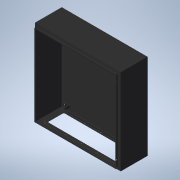
# Autodesk Inventor part: 1060.000(2)_P1
Saved by Autodesk Inventor 2021 (Build 250183000, 183)
## iProperties
Created: 2025-09-22
Part Number: 1060.000(2)_P1
Material: Generic
Catalog Web Link: www.cadenas.de
Description: AE 2.0 Gehaeuse-AE 2.0 Gehaeuse
Vendor: RITTAL
Document SubType Name: Modeling
Designer: psAdmin
Manufacturer: RITTAL
Mass: 1295.88 g
Surface Area: 17146.7 cm^2
Volume: 1295.88 cm^3
Density: 1 g/cm^3
Appearance: PSOLRGB-176-176-176
Category: PARTsolutions
Company: RITTAL
Title: 1060.000(2)_P1
Author: Cadenas PARTsolutions
Comments: AE 2.0 Gehaeuse
PSOL_IDENT_0: {$CADENAS_DATA/23d-libs/rittal/schaltschranksys/kompakt_schaltschr/parts_ae_2_0/gehaeuse_ae_2_0.prj}
PSOL_IDENT_1: ,190 {VTYP=3D},{NB=1060.000(2)_P1},{LINA=1060.000(2)_P1},{NN=AE 2.0 Gehaeuse},{DATE=25.07.2025 12:41
PSOL_IDENT_2: :23},{GEOMDATE=24.07.2025 05:50:00},{VERSION=},{LINEID=350},{WBVAR=DETAIL},{WBNUMERIC=DETAIL}  {NB=1
PSOL_IDENT_3: 060.000(2)_P1},{LINA=1060.000(2)_P1},{KT=DUMMY},{DETAIL=2},{BEZ1=Neues Kompaktgehäuse},{BEZ2=Stahlbl
PSOL_IDENT_4: ech},{BEZ3=eintürig},{TUER=1},{B=600},{H=600},{T=210},{F=550},{G=575},{B1=600},{BEST=1060.000},{B3=5
PSOL_IDENT_5: 60.000},{B4=470.000},{B5=498.000},{BB5=0.000},{H1=600},{H3=560.000},{H4=85.000},{H5=113.000},{HH5=4.
PSOL_IDENT_6: 000},{T5=93.500},{R1=31.000},{R2=8.000},{T1=210},{F1=550},{G1=575},{VERS3=0},{VERS=7},{CNSECLASS51=2
PSOL_IDENT_7: 7-18-01-02},{CNSECLASS70=27-18-01-01},{CNSECLASS80=27-18-01-01},{CNSETIM40=EC000261},{S=1.50},{W=600
PSOL_IDENT_8: .000},{W1=556.000},{W2=500.000},{HH=600.000},{HH1=556.000},{HH2=550.000},{HH3=475.000},{D=187.500},{
PSOL_IDENT_9: D1=205.100},{VERS1=1},{GEW=22,3},{CNSETIM80=EC000261},{CNSETIM90=EC000261},{CNSECLASS60=27-18-01-01}
PSOL_IDENT_10: ,{UNSPSC=31-26-15-02}
NB: 1060.000(2)_P1
NN: AE 2.0 Gehaeuse
NT: AE 2.0 Gehaeuse
NBSYN: $BEST.($DETAIL.)_P1
LINA: 1060.000(2)_P1
CATALOG: Rittal
DETAIL: niedrig
BEZ1: Neues Kompaktgehäuse
BEZ2: Stahlblech
BEZ3: eintürig
TUER: 1
B: 600
H: 600
T: 210
F: 550
G: 575
B1: 600
BEST: 1060.000
B3: 560
B4: 470
B5: 498
BB5: 0
H1: 600
H3: 560
H4: 85
H5: 113
HH5: 4
T5: 93.5
R1: 31
R2: 8
T1: 210
F1: 550
G1: 575
VERS3: 0
VERS: 7
CNSECLASS70: 27-18-01-01
CNSECLASS80: 27-18-01-01
S: 1.5
W: 600
W1: 556
W2: 500
HH: 600
HH1: 556
HH2: 550
HH3: 475
D: 187.5
D1: 205.1
VERS1: 1
GEW: 22,3
CNSETIM80: EC000261
CNSETIM90: EC000261
CNSECLASS60: 27-18-01-01
UNSPSC: 31-26-15-02
SUPPLIER: RITTAL
ARTICLENO: 1060.000(2)_P1
BOMINFO: 1060.000(2)_P1
CREATOR: CADENAS GmbH
Autodesk Inventor part; units mm, degrees
(part 1 of 2)
sketch "Sketch_1" plane through (0, 0, 0) normal (0, 1, 0) x (1, 0, 0)
  line L0 (-300, -82.5) -> (300, -82.5)
  line L1 (300, -82.5) -> (300, 105)
  line L2 (300, 105) -> (-300, 105)
  line L3 (-300, 105) -> (-300, -82.5)
  line L4 (-298.5, -81) -> (298.5, -81)
  line L5 (298.5, -81) -> (298.5, 103.5)
  line L6 (298.5, 103.5) -> (-298.5, 103.5)
  line L7 (-298.5, 103.5) -> (-298.5, -81)
  constraints: 16 end point
extrude "Extrusion1" add sketch "Sketch_1" along normal blind 600
sketch "Sketch_2" plane through (0, 0, 82.5) normal (0, 0, 1) x (1, 0, 0)
  line L0 (-281, 19) -> (281, 19)
  line L1 (281, 19) -> (281, 581)
  line L2 (281, 581) -> (-281, 581)
  line L3 (-281, 581) -> (-281, 19)
  constraints: 8 end point
extrude "Extrusion2" cut sketch "Sketch_2" against normal blind 1.5
sketch "Sketch_3" plane through (0, 0, 0) normal (1, 0, 0) x (0, 0, -1)
  line L0 (-82.5, 590) -> (-81, 590)
  line L1 (-81, 590) -> (-81, 598.5)
  line L2 (-81, 598.5) -> (103.5, 598.5)
  line L3 (103.5, 598.5) -> (103.5, 1.5)
  line L4 (103.5, 1.5) -> (-81, 1.5)
  line L5 (-81, 1.5) -> (-81, 10)
  line L6 (-81, 10) -> (-82.5, 10)
  line L7 (-82.5, 10) -> (-82.5, 0)
  line L8 (-82.5, 0) -> (105, 0)
  line L9 (105, 0) -> (105, 600)
  line L10 (105, 600) -> (-82.5, 600)
  line L11 (-82.5, 600) -> (-82.5, 590)
  constraints: 24 end point
extrude "Extrusion3" add sketch "Sketch_3" along normal mid plane 600
sketch "Sketch_48" plane through (0, 0, -105) normal (0, 0, 1) x (1, 0, 0)
  line L0 (-295.5, 595.5) -> (-295.5, 4.5)
  line L1 (-295.5, 4.5) -> (295.5, 4.5)
  line L2 (295.5, 4.5) -> (295.5, 595.5)
  line L3 (295.5, 595.5) -> (-295.5, 595.5)
  constraints: 8 end point
extrude "Extrusion4" cut sketch "Sketch_48" along normal blind 1.5
sketch "Sketch_49" plane through (0, 0, -105) normal (0, 0, 1) x (1, 0, 0)
  line L0 (-295.5, 595.5) -> (-295.5, 4.5)
  line L1 (-295.5, 4.5) -> (295.5, 4.5)
  line L2 (295.5, 4.5) -> (295.5, 595.5)
  line L3 (295.5, 595.5) -> (-295.5, 595.5)
  line L4 (268.5, 8.5) -> (291.5, 8.5)
  line L5 (291.5, 8.5) -> (291.5, 31.5)
  line L6 (291.5, 31.5) -> (268.5, 31.5)
  line L7 (268.5, 31.5) -> (268.5, 8.5)
  line L8 (268.5, 568.5) -> (291.5, 568.5)
  line L9 (291.5, 568.5) -> (291.5, 591.5)
  line L10 (291.5, 591.5) -> (268.5, 591.5)
  line L11 (268.5, 591.5) -> (268.5, 568.5)
  line L12 (-291.5, 8.5) -> (-268.5, 8.5)
  line L13 (-268.5, 8.5) -> (-268.5, 31.5)
  line L14 (-268.5, 31.5) -> (-291.5, 31.5)
  line L15 (-291.5, 31.5) -> (-291.5, 8.5)
  line L16 (-291.5, 568.5) -> (-268.5, 568.5)
  line L17 (-268.5, 568.5) -> (-268.5, 591.5)
  line L18 (-268.5, 591.5) -> (-291.5, 591.5)
  line L19 (-291.5, 591.5) -> (-291.5, 568.5)
  constraints: 40 end point
extrude "Extrusion5" add sketch "Sketch_49" along normal blind 1.5
sketch "Sketch_50" plane through (0, 20, 0) normal (0, 1, 0) x (1, 0, 0)
  line L0 (-291.5, 103.5) -> (-290.1732, 103.5)
  line L1 (-290.1732, 103.5) -> (-289.0185, 101.5)
  line L2 (-289.0185, 101.5) -> (-270.9815, 101.5)
  line L3 (-270.9815, 101.5) -> (-269.8268, 103.5)
  line L4 (-269.8268, 103.5) -> (-268.5, 103.5)
  line L5 (-268.5, 103.5) -> (-268.5, 105)
  line L6 (-268.5, 105) -> (-270, 105)
  line L7 (-270, 105) -> (-271.1547, 103)
  line L8 (-271.1547, 103) -> (-288.8453, 103)
  line L9 (-288.8453, 103) -> (-290, 105)
  line L10 (-290, 105) -> (-291.5, 105)
  line L11 (-291.5, 105) -> (-291.5, 103.5)
  constraints: 24 end point
extrude "Extrusion6" add sketch "Sketch_50" along normal mid plane 15.35
sketch "Sketch_51" plane through (0, 20, 0) normal (0, 1, 0) x (1, 0, 0)
  line L0 (268.5, 103.5) -> (269.8268, 103.5)
  line L1 (269.8268, 103.5) -> (270.9815, 101.5)
  line L2 (270.9815, 101.5) -> (289.0185, 101.5)
  line L3 (289.0185, 101.5) -> (290.1732, 103.5)
  line L4 (290.1732, 103.5) -> (291.5, 103.5)
  line L5 (291.5, 103.5) -> (291.5, 105)
  line L6 (291.5, 105) -> (290, 105)
  line L7 (290, 105) -> (288.8453, 103)
  line L8 (288.8453, 103) -> (271.1547, 103)
  line L9 (271.1547, 103) -> (270, 105)
  line L10 (270, 105) -> (268.5, 105)
  line L11 (268.5, 105) -> (268.5, 103.5)
  constraints: 24 end point
extrude "Extrusion7" add sketch "Sketch_51" along normal mid plane 15.35
sketch "Sketch_52" plane through (0, 27.675, 0) normal (0, 1, 0) x (1, 0, 0)
  line L0 (-272.325, 101.5) -> (-272.325, 103)
  line L1 (-272.325, 103) -> (-271.1547, 103)
  line L2 (-271.1547, 103) -> (-270, 105)
  line L3 (-270, 105) -> (-265.5, 105)
  line L4 (-265.5, 105) -> (-265.5, 103.5)
  line L5 (-265.5, 103.5) -> (-269.8268, 103.5)
  line L6 (-269.8268, 103.5) -> (-270.9815, 101.5)
  line L7 (-270.9815, 101.5) -> (-272.325, 101.5)
  line L8 (-272.325, 101.5) -> (-272.325, 103)
  constraints: 18 end point
revolve "Revolution1" add sketch "Sketch_52" angle 90 about axis through (-272.325, 27.675, -101.5) along (0, 0, 1)
sketch "Sketch_53" plane through (0, 27.675, 0) normal (0, 1, 0) x (1, 0, 0)
  line L0 (-287.675, 103) -> (-287.675, 101.5)
  line L1 (-287.675, 101.5) -> (-289.0185, 101.5)
  line L2 (-289.0185, 101.5) -> (-290.1732, 103.5)
  line L3 (-290.1732, 103.5) -> (-294.5, 103.5)
  line L4 (-294.5, 103.5) -> (-294.5, 105)
  line L5 (-294.5, 105) -> (-290, 105)
  line L6 (-290, 105) -> (-288.8453, 103)
  line L7 (-288.8453, 103) -> (-287.675, 103)
  line L8 (-287.675, 103) -> (-287.675, 101.5)
  constraints: 18 end point
revolve "Revolution2" add sketch "Sketch_53" angle 90 about axis through (-287.675, 27.675, -103) along (0, 0, -1)
sketch "Sketch_54" plane through (0, 27.675, 0) normal (0, 1, 0) x (1, 0, 0)
  line L0 (287.675, 101.5) -> (287.675, 103)
  line L1 (287.675, 103) -> (288.8453, 103)
  line L2 (288.8453, 103) -> (290, 105)
  line L3 (290, 105) -> (294.5, 105)
  line L4 (294.5, 105) -> (294.5, 103.5)
  line L5 (294.5, 103.5) -> (290.1732, 103.5)
  line L6 (290.1732, 103.5) -> (289.0185, 101.5)
  line L7 (289.0185, 101.5) -> (287.675, 101.5)
  line L8 (287.675, 101.5) -> (287.675, 103)
  constraints: 18 end point
revolve "Revolution3" add sketch "Sketch_54" angle 90 about axis through (287.675, 27.675, -101.5) along (0, 0, 1)
sketch "Sketch_55" plane through (0, 27.675, 0) normal (0, 1, 0) x (1, 0, 0)
  line L0 (272.325, 103) -> (272.325, 101.5)
  line L1 (272.325, 101.5) -> (270.9815, 101.5)
  line L2 (270.9815, 101.5) -> (269.8268, 103.5)
  line L3 (269.8268, 103.5) -> (265.5, 103.5)
  line L4 (265.5, 103.5) -> (265.5, 105)
  line L5 (265.5, 105) -> (270, 105)
  line L6 (270, 105) -> (271.1547, 103)
  line L7 (271.1547, 103) -> (272.325, 103)
  line L8 (272.325, 103) -> (272.325, 101.5)
  constraints: 18 end point
revolve "Revolution4" add sketch "Sketch_55" angle 90 about axis through (272.325, 27.675, -103) along (0, 0, -1)
sketch "Sketch_56" plane through (0, 12.325, 0) normal (0, 1, 0) x (1, 0, 0)
  line L0 (-272.325, 101.5) -> (-272.325, 103)
  line L1 (-272.325, 103) -> (-271.1547, 103)
  line L2 (-271.1547, 103) -> (-270, 105)
  line L3 (-270, 105) -> (-265.5, 105)
  line L4 (-265.5, 105) -> (-265.5, 103.5)
  line L5 (-265.5, 103.5) -> (-269.8268, 103.5)
  line L6 (-269.8268, 103.5) -> (-270.9815, 101.5)
  line L7 (-270.9815, 101.5) -> (-272.325, 101.5)
  line L8 (-272.325, 101.5) -> (-272.325, 103)
  constraints: 18 end point
revolve "Revolution5" add sketch "Sketch_56" angle 90 about axis through (-272.325, 12.325, -101.5) along (0, 0, -1)
sketch "Sketch_57" plane through (0, 12.325, 0) normal (0, 1, 0) x (1, 0, 0)
  line L0 (-287.675, 103) -> (-287.675, 101.5)
  line L1 (-287.675, 101.5) -> (-289.0185, 101.5)
  line L2 (-289.0185, 101.5) -> (-290.1732, 103.5)
  line L3 (-290.1732, 103.5) -> (-294.5, 103.5)
  line L4 (-294.5, 103.5) -> (-294.5, 105)
  line L5 (-294.5, 105) -> (-290, 105)
  line L6 (-290, 105) -> (-288.8453, 103)
  line L7 (-288.8453, 103) -> (-287.675, 103)
  line L8 (-287.675, 103) -> (-287.675, 101.5)
  constraints: 18 end point
revolve "Revolution6" add sketch "Sketch_57" angle 90 about axis through (-287.675, 12.325, -103) along (0, 0, 1)
sketch "Sketch_58" plane through (0, 12.325, 0) normal (0, 1, 0) x (1, 0, 0)
  line L0 (287.675, 101.5) -> (287.675, 103)
  line L1 (287.675, 103) -> (288.8453, 103)
  line L2 (288.8453, 103) -> (290, 105)
  line L3 (290, 105) -> (294.5, 105)
  line L4 (294.5, 105) -> (294.5, 103.5)
  line L5 (294.5, 103.5) -> (290.1732, 103.5)
  line L6 (290.1732, 103.5) -> (289.0185, 101.5)
  line L7 (289.0185, 101.5) -> (287.675, 101.5)
  line L8 (287.675, 101.5) -> (287.675, 103)
  constraints: 18 end point
revolve "Revolution7" add sketch "Sketch_58" angle 90 about axis through (287.675, 12.325, -101.5) along (0, 0, -1)
sketch "Sketch_59" plane through (0, 12.325, 0) normal (0, 1, 0) x (1, 0, 0)
  line L0 (272.325, 103) -> (272.325, 101.5)
  line L1 (272.325, 101.5) -> (270.9815, 101.5)
  line L2 (270.9815, 101.5) -> (269.8268, 103.5)
  line L3 (269.8268, 103.5) -> (265.5, 103.5)
  line L4 (265.5, 103.5) -> (265.5, 105)
  line L5 (265.5, 105) -> (270, 105)
  line L6 (270, 105) -> (271.1547, 103)
  line L7 (271.1547, 103) -> (272.325, 103)
  line L8 (272.325, 103) -> (272.325, 101.5)
  constraints: 18 end point
revolve "Revolution8" add sketch "Sketch_59" angle 90 about axis through (272.325, 12.325, -103) along (0, 0, 1)
sketch "Sketch_60" plane through (0, 580, 0) normal (0, 1, 0) x (1, 0, 0)
  line L0 (-291.5, 103.5) -> (-290.1732, 103.5)
  line L1 (-290.1732, 103.5) -> (-289.0185, 101.5)
  line L2 (-289.0185, 101.5) -> (-270.9815, 101.5)
  line L3 (-270.9815, 101.5) -> (-269.8268, 103.5)
  line L4 (-269.8268, 103.5) -> (-268.5, 103.5)
  line L5 (-268.5, 103.5) -> (-268.5, 105)
  line L6 (-268.5, 105) -> (-270, 105)
  line L7 (-270, 105) -> (-271.1547, 103)
  line L8 (-271.1547, 103) -> (-288.8453, 103)
  line L9 (-288.8453, 103) -> (-290, 105)
  line L10 (-290, 105) -> (-291.5, 105)
  line L11 (-291.5, 105) -> (-291.5, 103.5)
  constraints: 24 end point
extrude "Extrusion8" add sketch "Sketch_60" along normal mid plane 15.35
sketch "Sketch_61" plane through (0, 580, 0) normal (0, 1, 0) x (1, 0, 0)
  line L0 (268.5, 103.5) -> (269.8268, 103.5)
  line L1 (269.8268, 103.5) -> (270.9815, 101.5)
  line L2 (270.9815, 101.5) -> (289.0185, 101.5)
  line L3 (289.0185, 101.5) -> (290.1732, 103.5)
  line L4 (290.1732, 103.5) -> (291.5, 103.5)
  line L5 (291.5, 103.5) -> (291.5, 105)
  line L6 (291.5, 105) -> (290, 105)
  line L7 (290, 105) -> (288.8453, 103)
  line L8 (288.8453, 103) -> (271.1547, 103)
  line L9 (271.1547, 103) -> (270, 105)
  line L10 (270, 105) -> (268.5, 105)
  line L11 (268.5, 105) -> (268.5, 103.5)
  constraints: 24 end point
extrude "Extrusion9" add sketch "Sketch_61" along normal mid plane 15.35
sketch "Sketch_62" plane through (0, 587.675, 0) normal (0, 1, 0) x (1, 0, 0)
  line L0 (-272.325, 101.5) -> (-272.325, 103)
  line L1 (-272.325, 103) -> (-271.1547, 103)
  line L2 (-271.1547, 103) -> (-270, 105)
  line L3 (-270, 105) -> (-265.5, 105)
  line L4 (-265.5, 105) -> (-265.5, 103.5)
  line L5 (-265.5, 103.5) -> (-269.8268, 103.5)
  line L6 (-269.8268, 103.5) -> (-270.9815, 101.5)
  line L7 (-270.9815, 101.5) -> (-272.325, 101.5)
  line L8 (-272.325, 101.5) -> (-272.325, 103)
  constraints: 18 end point
revolve "Revolution9" add sketch "Sketch_62" angle 90 about axis through (-272.325, 587.675, -101.5) along (0, 0, 1)
sketch "Sketch_63" plane through (0, 587.675, 0) normal (0, 1, 0) x (1, 0, 0)
  line L0 (-287.675, 103) -> (-287.675, 101.5)
  line L1 (-287.675, 101.5) -> (-289.0185, 101.5)
  line L2 (-289.0185, 101.5) -> (-290.1732, 103.5)
  line L3 (-290.1732, 103.5) -> (-294.5, 103.5)
  line L4 (-294.5, 103.5) -> (-294.5, 105)
  line L5 (-294.5, 105) -> (-290, 105)
  line L6 (-290, 105) -> (-288.8453, 103)
  line L7 (-288.8453, 103) -> (-287.675, 103)
  line L8 (-287.675, 103) -> (-287.675, 101.5)
  constraints: 18 end point
revolve "Revolution10" add sketch "Sketch_63" angle 90 about axis through (-287.675, 587.675, -103) along (0, 0, -1)
sketch "Sketch_64" plane through (0, 587.675, 0) normal (0, 1, 0) x (1, 0, 0)
  line L0 (287.675, 101.5) -> (287.675, 103)
  line L1 (287.675, 103) -> (288.8453, 103)
  line L2 (288.8453, 103) -> (290, 105)
  line L3 (290, 105) -> (294.5, 105)
  line L4 (294.5, 105) -> (294.5, 103.5)
  line L5 (294.5, 103.5) -> (290.1732, 103.5)
  line L6 (290.1732, 103.5) -> (289.0185, 101.5)
  line L7 (289.0185, 101.5) -> (287.675, 101.5)
  line L8 (287.675, 101.5) -> (287.675, 103)
  constraints: 18 end point
revolve "Revolution11" add sketch "Sketch_64" angle 90 about axis through (287.675, 587.675, -101.5) along (0, 0, 1)
sketch "Sketch_65" plane through (0, 587.675, 0) normal (0, 1, 0) x (1, 0, 0)
  line L0 (272.325, 103) -> (272.325, 101.5)
  line L1 (272.325, 101.5) -> (270.9815, 101.5)
  line L2 (270.9815, 101.5) -> (269.8268, 103.5)
  line L3 (269.8268, 103.5) -> (265.5, 103.5)
  line L4 (265.5, 103.5) -> (265.5, 105)
  line L5 (265.5, 105) -> (270, 105)
  line L6 (270, 105) -> (271.1547, 103)
  line L7 (271.1547, 103) -> (272.325, 103)
  line L8 (272.325, 103) -> (272.325, 101.5)
  constraints: 18 end point
revolve "Revolution12" add sketch "Sketch_65" angle 90 about axis through (272.325, 587.675, -103) along (0, 0, -1)
sketch "Sketch_66" plane through (0, 572.325, 0) normal (0, 1, 0) x (1, 0, 0)
  line L0 (-272.325, 101.5) -> (-272.325, 103)
  line L1 (-272.325, 103) -> (-271.1547, 103)
  line L2 (-271.1547, 103) -> (-270, 105)
  line L3 (-270, 105) -> (-265.5, 105)
  line L4 (-265.5, 105) -> (-265.5, 103.5)
  line L5 (-265.5, 103.5) -> (-269.8268, 103.5)
  line L6 (-269.8268, 103.5) -> (-270.9815, 101.5)
  line L7 (-270.9815, 101.5) -> (-272.325, 101.5)
  line L8 (-272.325, 101.5) -> (-272.325, 103)
  constraints: 18 end point
revolve "Revolution13" add sketch "Sketch_66" angle 90 about axis through (-272.325, 572.325, -101.5) along (0, 0, -1)
sketch "Sketch_67" plane through (0, 572.325, 0) normal (0, 1, 0) x (1, 0, 0)
  line L0 (-287.675, 103) -> (-287.675, 101.5)
  line L1 (-287.675, 101.5) -> (-289.0185, 101.5)
  line L2 (-289.0185, 101.5) -> (-290.1732, 103.5)
  line L3 (-290.1732, 103.5) -> (-294.5, 103.5)
  line L4 (-294.5, 103.5) -> (-294.5, 105)
  line L5 (-294.5, 105) -> (-290, 105)
  line L6 (-290, 105) -> (-288.8453, 103)
  line L7 (-288.8453, 103) -> (-287.675, 103)
  line L8 (-287.675, 103) -> (-287.675, 101.5)
  constraints: 18 end point
revolve "Revolution14" add sketch "Sketch_67" angle 90 about axis through (-287.675, 572.325, -103) along (0, 0, 1)
sketch "Sketch_68" plane through (0, 572.325, 0) normal (0, 1, 0) x (1, 0, 0)
  line L0 (287.675, 101.5) -> (287.675, 103)
  line L1 (287.675, 103) -> (288.8453, 103)
  line L2 (288.8453, 103) -> (290, 105)
  line L3 (290, 105) -> (294.5, 105)
  line L4 (294.5, 105) -> (294.5, 103.5)
  line L5 (294.5, 103.5) -> (290.1732, 103.5)
  line L6 (290.1732, 103.5) -> (289.0185, 101.5)
  line L7 (289.0185, 101.5) -> (287.675, 101.5)
  line L8 (287.675, 101.5) -> (287.675, 103)
  constraints: 18 end point
revolve "Revolution15" add sketch "Sketch_68" angle 90 about axis through (287.675, 572.325, -101.5) along (0, 0, -1)
sketch "Sketch_69" plane through (0, 572.325, 0) normal (0, 1, 0) x (1, 0, 0)
  line L0 (272.325, 103) -> (272.325, 101.5)
  line L1 (272.325, 101.5) -> (270.9815, 101.5)
  line L2 (270.9815, 101.5) -> (269.8268, 103.5)
  line L3 (269.8268, 103.5) -> (265.5, 103.5)
  line L4 (265.5, 103.5) -> (265.5, 105)
  line L5 (265.5, 105) -> (270, 105)
  line L6 (270, 105) -> (271.1547, 103)
  line L7 (271.1547, 103) -> (272.325, 103)
  line L8 (272.325, 103) -> (272.325, 101.5)
  constraints: 18 end point
revolve "Revolution16" add sketch "Sketch_69" angle 90 about axis through (272.325, 572.325, -103) along (0, 0, 1)
sketch "Sketch_70" plane through (-280, 0, 0) normal (1, 0, 0) x (0, 0, -1)
  line L0 (101.5, 10.9815) -> (103.5, 9.8268)
  line L1 (103.5, 9.8268) -> (103.5, 8.5)
  line L2 (103.5, 8.5) -> (105, 8.5)
  line L3 (105, 8.5) -> (105, 10)
  line L4 (105, 10) -> (103, 11.1547)
  line L5 (103, 11.1547) -> (103, 28.8453)
  line L6 (103, 28.8453) -> (105, 30)
  line L7 (105, 30) -> (105, 31.5)
  line L8 (105, 31.5) -> (103.5, 31.5)
  line L9 (103.5, 31.5) -> (103.5, 30.1732)
  line L10 (103.5, 30.1732) -> (101.5, 29.0185)
  line L11 (101.5, 29.0185) -> (101.5, 10.9815)
  constraints: 24 end point
extrude "Extrusion10" add sketch "Sketch_70" along normal mid plane 15.35
sketch "Sketch_71" plane through (-280, 0, 0) normal (1, 0, 0) x (0, 0, -1)
  line L0 (101.5, 570.9815) -> (103.5, 569.8268)
  line L1 (103.5, 569.8268) -> (103.5, 568.5)
  line L2 (103.5, 568.5) -> (105, 568.5)
  line L3 (105, 568.5) -> (105, 570)
  line L4 (105, 570) -> (103, 571.1547)
  line L5 (103, 571.1547) -> (103, 588.8453)
  line L6 (103, 588.8453) -> (105, 590)
  line L7 (105, 590) -> (105, 591.5)
  line L8 (105, 591.5) -> (103.5, 591.5)
  line L9 (103.5, 591.5) -> (103.5, 590.1732)
  line L10 (103.5, 590.1732) -> (101.5, 589.0185)
  line L11 (101.5, 589.0185) -> (101.5, 570.9815)
  constraints: 24 end point
extrude "Extrusion11" add sketch "Sketch_71" along normal mid plane 15.35
sketch "Sketch_74" plane through (-280, 0, 0) normal (1, 0, 0) x (0, 0, -1)
  line L0 (104.5, 20) -> (101.5, 20)
  line L1 (101.5, 20) -> (101.5, 26.25)
  line L2 (101.5, 26.25) -> (103, 26.25)
  line L3 (103, 26.25) -> (103, 25.6)
  line L4 (103, 25.6) -> (104.5, 25.6)
  line L5 (104.5, 25.6) -> (104.5, 20)
  line L6 (104.5, 20) -> (101.5, 20)
  constraints: 14 end point
revolve "Revolution17" add sketch "Sketch_74" angle 360 about axis through (-280, 20, -104.5) along (0, 0, 1)
sketch "Sketch_75" plane through (-280, 0, 0) normal (1, 0, 0) x (0, 0, -1)
  line L0 (105, 20) -> (101, 20)
  line L1 (101, 20) -> (101, 25.625)
  line L2 (101, 25.625) -> (101.5, 25.625)
  line L3 (101.5, 25.625) -> (101.5, 24.625)
  line L4 (101.5, 24.625) -> (104.5, 24.625)
  line L5 (104.5, 24.625) -> (104.5, 25.625)
  line L6 (104.5, 25.625) -> (105, 25.625)
  line L7 (105, 25.625) -> (105, 20)
  line L8 (105, 20) -> (101, 20)
  constraints: 18 end point
revolve "Revolution18" cut sketch "Sketch_75" angle 360 about axis through (-280, 20, -105) along (0, 0, 1)
sketch "Sketch_76" plane through (-280, 0, 0) normal (1, 0, 0) x (0, 0, -1)
  line L0 (104.5, 580) -> (101.5, 580)
  line L1 (101.5, 580) -> (101.5, 586.25)
  line L2 (101.5, 586.25) -> (103, 586.25)
  line L3 (103, 586.25) -> (103, 585.6)
  line L4 (103, 585.6) -> (104.5, 585.6)
  line L5 (104.5, 585.6) -> (104.5, 580)
  line L6 (104.5, 580) -> (101.5, 580)
  constraints: 14 end point
revolve "Revolution19" add sketch "Sketch_76" angle 360 about axis through (-280, 580, -104.5) along (0, 0, 1)
sketch "Sketch_77" plane through (-280, 0, 0) normal (1, 0, 0) x (0, 0, -1)
  line L0 (105, 580) -> (101, 580)
  line L1 (101, 580) -> (101, 585.625)
  line L2 (101, 585.625) -> (101.5, 585.625)
  line L3 (101.5, 585.625) -> (101.5, 584.625)
  line L4 (101.5, 584.625) -> (104.5, 584.625)
  line L5 (104.5, 584.625) -> (104.5, 585.625)
  line L6 (104.5, 585.625) -> (105, 585.625)
  line L7 (105, 585.625) -> (105, 580)
  line L8 (105, 580) -> (101, 580)
  constraints: 18 end point
revolve "Revolution20" cut sketch "Sketch_77" angle 360 about axis through (-280, 580, -105) along (0, 0, 1)
sketch "Sketch_72" plane through (280, 0, 0) normal (1, 0, 0) x (0, 0, -1)
  line L0 (101.5, 10.9815) -> (103.5, 9.8268)
  line L1 (103.5, 9.8268) -> (103.5, 8.5)
  line L2 (103.5, 8.5) -> (105, 8.5)
  line L3 (105, 8.5) -> (105, 10)
  line L4 (105, 10) -> (103, 11.1547)
  line L5 (103, 11.1547) -> (103, 28.8453)
  line L6 (103, 28.8453) -> (105, 30)
  line L7 (105, 30) -> (105, 31.5)
  line L8 (105, 31.5) -> (103.5, 31.5)
  line L9 (103.5, 31.5) -> (103.5, 30.1732)
  line L10 (103.5, 30.1732) -> (101.5, 29.0185)
  line L11 (101.5, 29.0185) -> (101.5, 10.9815)
  constraints: 24 end point
extrude "Extrusion12" add sketch "Sketch_72" along normal mid plane 15.35
sketch "Sketch_73" plane through (280, 0, 0) normal (1, 0, 0) x (0, 0, -1)
  line L0 (101.5, 570.9815) -> (103.5, 569.8268)
  line L1 (103.5, 569.8268) -> (103.5, 568.5)
  line L2 (103.5, 568.5) -> (105, 568.5)
  line L3 (105, 568.5) -> (105, 570)
  line L4 (105, 570) -> (103, 571.1547)
  line L5 (103, 571.1547) -> (103, 588.8453)
  line L6 (103, 588.8453) -> (105, 590)
  line L7 (105, 590) -> (105, 591.5)
  line L8 (105, 591.5) -> (103.5, 591.5)
  line L9 (103.5, 591.5) -> (103.5, 590.1732)
  line L10 (103.5, 590.1732) -> (101.5, 589.0185)
  line L11 (101.5, 589.0185) -> (101.5, 570.9815)
  constraints: 24 end point
extrude "Extrusion13" add sketch "Sketch_73" along normal mid plane 15.35
sketch "Sketch_78" plane through (280, 0, 0) normal (1, 0, 0) x (0, 0, -1)
  line L0 (104.5, 20) -> (101.5, 20)
  line L1 (101.5, 20) -> (101.5, 26.25)
  line L2 (101.5, 26.25) -> (103, 26.25)
  line L3 (103, 26.25) -> (103, 25.6)
  line L4 (103, 25.6) -> (104.5, 25.6)
  line L5 (104.5, 25.6) -> (104.5, 20)
  line L6 (104.5, 20) -> (101.5, 20)
  constraints: 14 end point
revolve "Revolution21" add sketch "Sketch_78" angle 360 about axis through (280, 20, -104.5) along (0, 0, 1)
sketch "Sketch_79" plane through (280, 0, 0) normal (1, 0, 0) x (0, 0, -1)
  line L0 (105, 20) -> (101, 20)
  line L1 (101, 20) -> (101, 25.625)
  line L2 (101, 25.625) -> (101.5, 25.625)
  line L3 (101.5, 25.625) -> (101.5, 24.625)
  line L4 (101.5, 24.625) -> (104.5, 24.625)
  line L5 (104.5, 24.625) -> (104.5, 25.625)
  line L6 (104.5, 25.625) -> (105, 25.625)
  line L7 (105, 25.625) -> (105, 20)
  line L8 (105, 20) -> (101, 20)
  constraints: 18 end point
revolve "Revolution22" cut sketch "Sketch_79" angle 360 about axis through (280, 20, -105) along (0, 0, 1)
sketch "Sketch_80" plane through (280, 0, 0) normal (1, 0, 0) x (0, 0, -1)
  line L0 (104.5, 580) -> (101.5, 580)
  line L1 (101.5, 580) -> (101.5, 586.25)
  line L2 (101.5, 586.25) -> (103, 586.25)
  line L3 (103, 586.25) -> (103, 585.6)
  line L4 (103, 585.6) -> (104.5, 585.6)
  line L5 (104.5, 585.6) -> (104.5, 580)
  line L6 (104.5, 580) -> (101.5, 580)
  constraints: 14 end point
revolve "Revolution23" add sketch "Sketch_80" angle 360 about axis through (280, 580, -104.5) along (0, 0, 1)
sketch "Sketch_81" plane through (280, 0, 0) normal (1, 0, 0) x (0, 0, -1)
  line L0 (105, 580) -> (101, 580)
  line L1 (101, 580) -> (101, 585.625)
  line L2 (101, 585.625) -> (101.5, 585.625)
  line L3 (101.5, 585.625) -> (101.5, 584.625)
  line L4 (101.5, 584.625) -> (104.5, 584.625)
  line L5 (104.5, 584.625) -> (104.5, 585.625)
  line L6 (104.5, 585.625) -> (105, 585.625)
  line L7 (105, 585.625) -> (105, 580)
  line L8 (105, 580) -> (101, 580)
  constraints: 18 end point
revolve "Revolution24" cut sketch "Sketch_81" angle 360 about axis through (280, 580, -105) along (0, 0, 1)
sketch "Sketch_6" plane through (0, 0, 0) normal (1, 0, 0) x (0, 0, -1)
  line L0 (-100.1, 585.9693) -> (-99.4028, 578)
  line L1 (-99.4028, 578) -> (-81, 578)
  line L2 (-81, 578) -> (-81, 586.1)
  line L3 (-81, 586.1) -> (-98.6057, 586.1)
  line L4 (-98.6057, 586.1) -> (-100.1, 585.9693)
  constraints: 10 end point
extrude "Extrusion14" add sketch "Sketch_6" along normal mid plane 574.2
sketch "Sketch_7" plane through (0, 0, 0) normal (1, 0, 0) x (0, 0, -1)
  line L0 (-100.1, 14.0307) -> (-98.6057, 13.9)
  line L1 (-98.6057, 13.9) -> (-81, 13.9)
  line L2 (-81, 13.9) -> (-81, 22)
  line L3 (-81, 22) -> (-99.4028, 22)
  line L4 (-99.4028, 22) -> (-100.1, 14.0307)
  constraints: 10 end point
extrude "Extrusion15" add sketch "Sketch_7" along normal mid plane 574.2
sketch "Sketch_8" plane through (0, 300, 0) normal (0, 1, 0) x (1, 0, 0)
  line L0 (278, -99.4028) -> (285.9693, -100.1)
  line L1 (285.9693, -100.1) -> (286.1, -98.6057)
  line L2 (286.1, -98.6057) -> (286.1, -81)
  line L3 (286.1, -81) -> (278, -81)
  line L4 (278, -81) -> (278, -99.4028)
  constraints: 10 end point
extrude "Extrusion16" add sketch "Sketch_8" along normal mid plane 574.2
sketch "Sketch_9" plane through (0, 300, 0) normal (0, 1, 0) x (1, 0, 0)
  line L0 (-286.1, -98.6057) -> (-285.9693, -100.1)
  line L1 (-285.9693, -100.1) -> (-278, -99.4028)
  line L2 (-278, -99.4028) -> (-278, -81)
  line L3 (-278, -81) -> (-286.1, -81)
  line L4 (-286.1, -81) -> (-286.1, -98.6057)
  constraints: 10 end point
extrude "Extrusion17" add sketch "Sketch_9" along normal mid plane 574.2
sketch "Sketch_10" plane through (0, 300, 0) normal (0, 1, 0) x (1, 0, 0)
  line L0 (-287.6, -82.5) -> (-287.6, -103.1)
  line L1 (-287.6, -103.1) -> (287.6, -103.1)
  line L2 (287.6, -103.1) -> (287.6, -82.5)
  line L3 (287.6, -82.5) -> (279.5, -82.5)
  line L4 (279.5, -82.5) -> (279.5, -98.0283)
  line L5 (279.5, -98.0283) -> (286.1, -98.6057)
  line L6 (286.1, -98.6057) -> (285.9693, -100.1)
  line L7 (285.9693, -100.1) -> (-285.9693, -100.1)
  line L8 (-285.9693, -100.1) -> (-286.1, -98.6057)
  line L9 (-286.1, -98.6057) -> (-279.5, -98.0283)
  line L10 (-279.5, -98.0283) -> (-279.5, -82.5)
  line L11 (-279.5, -82.5) -> (-287.6, -82.5)
  constraints: 24 end point
extrude "Extrusion18" cut sketch "Sketch_10" along normal mid plane 572.2
sketch "Sketch_11" plane through (0, 0, 0) normal (1, 0, 0) x (0, 0, -1)
  line L0 (-103.1, 10.9) -> (-82.5, 10.9)
  line L1 (-82.5, 10.9) -> (-82.5, 20.5)
  line L2 (-82.5, 20.5) -> (-98.0283, 20.5)
  line L3 (-98.0283, 20.5) -> (-98.6057, 13.9)
  line L4 (-98.6057, 13.9) -> (-100.1, 14.0307)
  line L5 (-100.1, 14.0307) -> (-100.1, 585.9693)
  line L6 (-100.1, 585.9693) -> (-98.6057, 586.1)
  line L7 (-98.6057, 586.1) -> (-98.0283, 579.5)
  line L8 (-98.0283, 579.5) -> (-82.5, 579.5)
  line L9 (-82.5, 579.5) -> (-82.5, 589.1)
  line L10 (-82.5, 589.1) -> (-103.1, 589.1)
  line L11 (-103.1, 589.1) -> (-103.1, 10.9)
  constraints: 24 end point
extrude "Extrusion19" cut sketch "Sketch_11" along normal mid plane 572.2
sketch "Sketch_13" plane through (0, 575, 0) normal (0, 1, 0) x (1, 0, 0)
  line L0 (-250, 72.5) -> (-250, 103.5)
  line L1 (-250, 103.5) -> (-243.5, 103.5)
  line L2 (-243.5, 103.5) -> (-243.5, 102.5)
  line L3 (-243.5, 102.5) -> (-242.45, 102.5)
  line L4 (-242.45, 102.5) -> (-242.25, 102.3)
  line L5 (-242.25, 102.3) -> (-242.25, 93.3)
  arc A0 (-242.55, 93) -> (-242.25, 93.3) centre (-242.55, 93.3) ccw
  line L6 (-242.55, 93) -> (-242.25, 93)
  line L7 (-242.25, 93) -> (-242.25, 87.5)
  line L8 (-242.25, 87.5) -> (-246, 87.5)
  line L9 (-246, 87.5) -> (-246, 85)
  line L10 (-246, 85) -> (-241, 85)
  arc A1 (-240.8875, 82.5051) -> (-241, 85) centre (-241, 83.75) ccw
  line L11 (-240.8875, 82.5051) -> (-242.2, 82.3864)
  line L12 (-242.2, 82.3864) -> (-242.2, 77.3483)
  line L13 (-242.2, 77.3483) -> (-243.5, 77)
  line L14 (-243.5, 77) -> (-246, 77)
  line L15 (-246, 77) -> (-246, 73.267)
  line L16 (-246, 73.267) -> (-246.767, 72.5)
  line L17 (-246.767, 72.5) -> (-250, 72.5)
  line L18 (-250, 72.5) -> (-250, 103.5)
  constraints: 38 end point, 4 point on circle, 2 centre point
revolve "Revolution25" add sketch "Sketch_13" angle 360 about axis through (-250, 575, -72.5) along (0, 0, 1)
thread "Thread1" size "M8x1.25" class "6g" standard "ISO Metric profile" length 1.1716
sketch "Sketch_14" plane through (0, 575, 0) normal (0, 1, 0) x (1, 0, 0)
  line L0 (250, 72.5) -> (250, 103.5)
  line L1 (250, 103.5) -> (256.5, 103.5)
  line L2 (256.5, 103.5) -> (256.5, 102.5)
  line L3 (256.5, 102.5) -> (257.55, 102.5)
  line L4 (257.55, 102.5) -> (257.75, 102.3)
  line L5 (257.75, 102.3) -> (257.75, 93.3)
  arc A0 (257.45, 93) -> (257.75, 93.3) centre (257.45, 93.3) ccw
  line L6 (257.45, 93) -> (257.75, 93)
  line L7 (257.75, 93) -> (257.75, 87.5)
  line L8 (257.75, 87.5) -> (254, 87.5)
  line L9 (254, 87.5) -> (254, 85)
  line L10 (254, 85) -> (259, 85)
  arc A1 (259.1125, 82.5051) -> (259, 85) centre (259, 83.75) ccw
  line L11 (259.1125, 82.5051) -> (257.8, 82.3864)
  line L12 (257.8, 82.3864) -> (257.8, 77.3483)
  line L13 (257.8, 77.3483) -> (256.5, 77)
  line L14 (256.5, 77) -> (254, 77)
  line L15 (254, 77) -> (254, 73.267)
  line L16 (254, 73.267) -> (253.233, 72.5)
  line L17 (253.233, 72.5) -> (250, 72.5)
  line L18 (250, 72.5) -> (250, 103.5)
  constraints: 38 end point, 4 point on circle, 2 centre point
revolve "Revolution26" add sketch "Sketch_14" angle 360 about axis through (250, 575, -72.5) along (0, 0, 1)
thread "Thread2" size "M8x1.25" class "6g" standard "ISO Metric profile" length 1.1716
sketch "Sketch_15" plane through (0, 25, 0) normal (0, 1, 0) x (1, 0, 0)
  line L0 (-250, 72.5) -> (-250, 103.5)
  line L1 (-250, 103.5) -> (-243.5, 103.5)
  line L2 (-243.5, 103.5) -> (-243.5, 102.5)
  line L3 (-243.5, 102.5) -> (-242.45, 102.5)
  line L4 (-242.45, 102.5) -> (-242.25, 102.3)
  line L5 (-242.25, 102.3) -> (-242.25, 93.3)
  arc A0 (-242.55, 93) -> (-242.25, 93.3) centre (-242.55, 93.3) ccw
  line L6 (-242.55, 93) -> (-242.25, 93)
  line L7 (-242.25, 93) -> (-242.25, 87.5)
  line L8 (-242.25, 87.5) -> (-246, 87.5)
  line L9 (-246, 87.5) -> (-246, 85)
  line L10 (-246, 85) -> (-241, 85)
  arc A1 (-240.8875, 82.5051) -> (-241, 85) centre (-241, 83.75) ccw
  line L11 (-240.8875, 82.5051) -> (-242.2, 82.3864)
  line L12 (-242.2, 82.3864) -> (-242.2, 77.3483)
  line L13 (-242.2, 77.3483) -> (-243.5, 77)
  line L14 (-243.5, 77) -> (-246, 77)
  line L15 (-246, 77) -> (-246, 73.267)
  line L16 (-246, 73.267) -> (-246.767, 72.5)
  line L17 (-246.767, 72.5) -> (-250, 72.5)
  line L18 (-250, 72.5) -> (-250, 103.5)
  constraints: 38 end point, 4 point on circle, 2 centre point
revolve "Revolution27" add sketch "Sketch_15" angle 360 about axis through (-250, 25, -72.5) along (0, 0, 1)
thread "Thread3" size "M8x1.25" class "6g" standard "ISO Metric profile" length 1.1716
sketch "Sketch_16" plane through (0, 25, 0) normal (0, 1, 0) x (1, 0, 0)
  line L0 (250, 72.5) -> (250, 103.5)
  line L1 (250, 103.5) -> (256.5, 103.5)
  line L2 (256.5, 103.5) -> (256.5, 102.5)
  line L3 (256.5, 102.5) -> (257.55, 102.5)
  line L4 (257.55, 102.5) -> (257.75, 102.3)
  line L5 (257.75, 102.3) -> (257.75, 93.3)
  arc A0 (257.45, 93) -> (257.75, 93.3) centre (257.45, 93.3) ccw
  line L6 (257.45, 93) -> (257.75, 93)
  line L7 (257.75, 93) -> (257.75, 87.5)
  line L8 (257.75, 87.5) -> (254, 87.5)
  line L9 (254, 87.5) -> (254, 85)
  line L10 (254, 85) -> (259, 85)
  arc A1 (259.1125, 82.5051) -> (259, 85) centre (259, 83.75) ccw
  line L11 (259.1125, 82.5051) -> (257.8, 82.3864)
  line L12 (257.8, 82.3864) -> (257.8, 77.3483)
  line L13 (257.8, 77.3483) -> (256.5, 77)
  line L14 (256.5, 77) -> (254, 77)
  line L15 (254, 77) -> (254, 73.267)
  line L16 (254, 73.267) -> (253.233, 72.5)
  line L17 (253.233, 72.5) -> (250, 72.5)
  line L18 (250, 72.5) -> (250, 103.5)
  constraints: 38 end point, 4 point on circle, 2 centre point
revolve "Revolution28" add sketch "Sketch_16" angle 360 about axis through (250, 25, -72.5) along (0, 0, 1)
thread "Thread4" size "M8x1.25" class "6g" standard "ISO Metric profile" length 1.1716
sketch "Sketch_100" plane through (0, 0, -76.75) normal (0, 0, 1) x (1, 0, 0)
  line L0 (-297, 597) -> (-297, 3)
  line L1 (-297, 3) -> (297, 3)
  line L2 (297, 3) -> (297, 597)
  line L3 (297, 597) -> (-297, 597)
  line L4 (243.5, 571.2472) -> (250, 567.4944)
  line L5 (250, 567.4944) -> (256.5, 571.2472)
  line L6 (256.5, 571.2472) -> (256.5, 578.7528)
  line L7 (256.5, 578.7528) -> (250, 582.5056)
  line L8 (250, 582.5056) -> (243.5, 578.7528)
  line L9 (243.5, 578.7528) -> (243.5, 571.2472)
  line L10 (243.5, 21.2472) -> (250, 17.4944)
  line L11 (250, 17.4944) -> (256.5, 21.2472)
  line L12 (256.5, 21.2472) -> (256.5, 28.7528)
  line L13 (256.5, 28.7528) -> (250, 32.5056)
  line L14 (250, 32.5056) -> (243.5, 28.7528)
  line L15 (243.5, 28.7528) -> (243.5, 21.2472)
  line L16 (-6.5, 571.2472) -> (0, 567.4944)
  line L17 (0, 567.4944) -> (6.5, 571.2472)
  line L18 (6.5, 571.2472) -> (6.5, 578.7528)
  line L19 (6.5, 578.7528) -> (0, 582.5056)
  line L20 (0, 582.5056) -> (-6.5, 578.7528)
  line L21 (-6.5, 578.7528) -> (-6.5, 571.2472)
  line L22 (-6.5, 21.2472) -> (0, 17.4944)
  line L23 (0, 17.4944) -> (6.5, 21.2472)
  line L24 (6.5, 21.2472) -> (6.5, 28.7528)
  line L25 (6.5, 28.7528) -> (0, 32.5056)
  line L26 (0, 32.5056) -> (-6.5, 28.7528)
  line L27 (-6.5, 28.7528) -> (-6.5, 21.2472)
  line L28 (-256.5, 571.2472) -> (-250, 567.4944)
  line L29 (-250, 567.4944) -> (-243.5, 571.2472)
  line L30 (-243.5, 571.2472) -> (-243.5, 578.7528)
  line L31 (-243.5, 578.7528) -> (-250, 582.5056)
  line L32 (-250, 582.5056) -> (-256.5, 578.7528)
  line L33 (-256.5, 578.7528) -> (-256.5, 571.2472)
  line L34 (-256.5, 21.2472) -> (-250, 17.4944)
  line L35 (-250, 17.4944) -> (-243.5, 21.2472)
  line L36 (-243.5, 21.2472) -> (-243.5, 28.7528)
  line L37 (-243.5, 28.7528) -> (-250, 32.5056)
  line L38 (-250, 32.5056) -> (-256.5, 28.7528)
  line L39 (-256.5, 28.7528) -> (-256.5, 21.2472)
  constraints: 80 end point
extrude "Extrusion20" cut sketch "Sketch_100" against normal blind 6
sketch "Sketch_139" plane through (0, 25, 0) normal (0, 1, 0) x (1, 0, 0)
  line L0 (-250, 81.6814) -> (-250, 85)
  line L1 (-250, 85) -> (-241, 85)
  arc A0 (-240.8875, 82.5051) -> (-241, 85) centre (-241, 83.75) ccw
  line L2 (-240.8875, 82.5051) -> (-250, 81.6814)
  line L3 (-250, 81.6814) -> (-250, 85)
  constraints: 8 end point, 2 point on circle, 1 centre point
revolve "Revolution29" add sketch "Sketch_139" angle 360 about axis through (-250, 25, -81.6814) along (0, 0, 1)
sketch "Sketch_140" plane through (0, 25, 0) normal (0, 1, 0) x (1, 0, 0)
  line L0 (250, 81.6814) -> (250, 85)
  line L1 (250, 85) -> (259, 85)
  arc A0 (259.1125, 82.5051) -> (259, 85) centre (259, 83.75) ccw
  line L2 (259.1125, 82.5051) -> (250, 81.6814)
  line L3 (250, 81.6814) -> (250, 85)
  constraints: 8 end point, 2 point on circle, 1 centre point
revolve "Revolution30" add sketch "Sketch_140" angle 360 about axis through (250, 25, -81.6814) along (0, 0, 1)
sketch "Sketch51" plane through (279.5, 20.5, 98.0283) normal (1, 0, 0) x (0, 0, -1)
  point P0 (8.2783, 517)
hole "Hole1" at (279.5, 537.5, 89.75) direction (-1, 0, 0) diameter 6.5 depth 1.5
sketch "Sketch52" plane through (279.5, 20.5, 98.0283) normal (1, 0, 0) x (0, 0, -1)
  point P0 (8.2783, 42)
hole "Hole2" at (279.5, 62.5, 89.75) direction (-1, 0, 0) diameter 6.5 depth 1.5
sketch "Sketch53" plane through (-279.5, 20.5, 82.5) normal (-1, 0, 0) x (0, 0, 1)
  point P0 (7.25, 517)
hole "Hole3" at (-279.5, 537.5, 89.75) direction (1, 0, 0) diameter 6.5 depth 1.5
sketch "Sketch54" plane through (-279.5, 20.5, 82.5) normal (-1, 0, 0) x (0, 0, 1)
  point P0 (7.25, 42)
hole "Hole4" at (-279.5, 62.5, 89.75) direction (1, 0, 0) diameter 6.5 depth 1.5
sketch "Sketch_27" plane through (0, 0, 0) normal (0, 1, 0) x (1, 0, 0)
  line L0 (-295.5, -78) -> (295.5, -78)
  line L1 (295.5, -78) -> (295.5, 100.5)
  line L2 (295.5, 100.5) -> (-295.5, 100.5)
  line L3 (-295.5, 100.5) -> (-295.5, -78)
  constraints: 8 end point
extrude "Extrusion21" cut sketch "Sketch_27" along normal blind 1.5
sketch "Sketch_28" plane through (0, 0, 0) normal (0, 1, 0) x (1, 0, 0)
  line L0 (-295.5, -78) -> (295.5, -78)
  line L1 (295.5, -78) -> (295.5, 100.5)
  line L2 (295.5, 100.5) -> (-295.5, 100.5)
  line L3 (-295.5, 100.5) -> (-295.5, -78)
  arc A0 (-274, -31) -> (-235, -70) centre (-235, -31) ccw
  line L4 (-235, -70) -> (235, -70)
  arc A1 (235, -70) -> (274, -31) centre (235, -31) ccw
  line L5 (274, -31) -> (274, 54)
  arc A2 (274, 54) -> (235, 93) centre (235, 54) ccw
  line L6 (235, 93) -> (-235, 93)
  arc A3 (-235, 93) -> (-274, 54) centre (-235, 54) ccw
  line L7 (-274, 54) -> (-274, -31)
  circle A4 centre (-283.5, -66) radius 8
  constraints: 16 end point, 8 point on circle, 5 centre point
extrude "Extrusion22" add sketch "Sketch_28" along normal blind 1.5
sketch "Sketch_29" plane through (0, 0, 0) normal (1, 0, 0) x (0, 0, -1)
  line L0 (68, 4) -> (84.5981, 4)
  line L1 (84.5981, 4) -> (91.5263, 0)
  line L2 (91.5263, 0) -> (93, 0)
  line L3 (93, 0) -> (93, 1.5)
  line L4 (93, 1.5) -> (91.9282, 1.5)
  line L5 (91.9282, 1.5) -> (85, 5.5)
  line L6 (85, 5.5) -> (68, 5.5)
  line L7 (68, 5.5) -> (68, 4)
  constraints: 16 end point
extrude "Extrusion23" add sketch "Sketch_29" along normal mid plane 470
sketch "Sketch_30" plane through (0, 0, 0) normal (1, 0, 0) x (0, 0, -1)
  line L0 (-70, 0) -> (-68.5263, 0)
  line L1 (-68.5263, 0) -> (-61.5981, 4)
  line L2 (-61.5981, 4) -> (-45, 4)
  line L3 (-45, 4) -> (-45, 5.5)
  line L4 (-45, 5.5) -> (-62, 5.5)
  line L5 (-62, 5.5) -> (-68.9282, 1.5)
  line L6 (-68.9282, 1.5) -> (-70, 1.5)
  line L7 (-70, 1.5) -> (-70, 0)
  constraints: 16 end point
extrude "Extrusion24" add sketch "Sketch_30" along normal mid plane 470
sketch "Sketch_31" plane through (235, 0, 0) normal (1, 0, 0) x (0, 0, -1)
  line L0 (54, 4) -> (54, 5.5)
  line L1 (68, 4) -> (84.5981, 4)
  line L2 (84.5981, 4) -> (91.5263, 0)
  line L3 (91.5263, 0) -> (95, 0)
  line L4 (95, 0) -> (95, 1.5)
  line L5 (95, 1.5) -> (91.9282, 1.5)
  line L6 (91.9282, 1.5) -> (85, 5.5)
  line L7 (85, 5.5) -> (68, 5.5)
  line L8 (68, 5.5) -> (68, 4)
  constraints: 18 end point
revolve "Revolution31" add sketch "Sketch_31" angle 90 about axis through (235, 4, -54) along (0, -1, 0)
sketch "Sketch_32" plane through (235, 0, 0) normal (1, 0, 0) x (0, 0, -1)
  line L0 (-31, 5.5) -> (-31, 4)
  line L1 (-72, 0) -> (-68.5263, 0)
  line L2 (-68.5263, 0) -> (-61.5981, 4)
  line L3 (-61.5981, 4) -> (-45, 4)
  line L4 (-45, 4) -> (-45, 5.5)
  line L5 (-45, 5.5) -> (-62, 5.5)
  line L6 (-62, 5.5) -> (-68.9282, 1.5)
  line L7 (-68.9282, 1.5) -> (-72, 1.5)
  line L8 (-72, 1.5) -> (-72, 0)
  constraints: 18 end point
revolve "Revolution32" add sketch "Sketch_32" angle 90 about axis through (235, 5.5, 31) along (0, 1, 0)
sketch "Sketch_33" plane through (-235, 0, 0) normal (1, 0, 0) x (0, 0, -1)
  line L0 (54, 4) -> (54, 5.5)
  line L1 (68, 4) -> (84.5981, 4)
  line L2 (84.5981, 4) -> (91.5263, 0)
  line L3 (91.5263, 0) -> (95, 0)
  line L4 (95, 0) -> (95, 1.5)
  line L5 (95, 1.5) -> (91.9282, 1.5)
  line L6 (91.9282, 1.5) -> (85, 5.5)
  line L7 (85, 5.5) -> (68, 5.5)
  line L8 (68, 5.5) -> (68, 4)
  constraints: 18 end point
revolve "Revolution33" add sketch "Sketch_33" angle 90 about axis through (-235, 4, -54) along (0, 1, 0)
sketch "Sketch_34" plane through (-235, 0, 0) normal (1, 0, 0) x (0, 0, -1)
  line L0 (-31, 5.5) -> (-31, 4)
  line L1 (-72, 0) -> (-68.5263, 0)
  line L2 (-68.5263, 0) -> (-61.5981, 4)
  line L3 (-61.5981, 4) -> (-45, 4)
  line L4 (-45, 4) -> (-45, 5.5)
  line L5 (-45, 5.5) -> (-62, 5.5)
  line L6 (-62, 5.5) -> (-68.9282, 1.5)
  line L7 (-68.9282, 1.5) -> (-72, 1.5)
  line L8 (-72, 1.5) -> (-72, 0)
  constraints: 18 end point
revolve "Revolution34" add sketch "Sketch_34" angle 90 about axis through (-235, 5.5, 31) along (0, -1, 0)
sketch "Sketch_35" plane through (0, 0, -11.5) normal (0, 0, 1) x (1, 0, 0)
  line L0 (249, 4) -> (265.5981, 4)
  line L1 (265.5981, 4) -> (272.5263, 0)
  line L2 (272.5263, 0) -> (274, 0)
  line L3 (274, 0) -> (274, 1.5)
  line L4 (274, 1.5) -> (272.9282, 1.5)
  line L5 (272.9282, 1.5) -> (266, 5.5)
  line L6 (266, 5.5) -> (249, 5.5)
  line L7 (249, 5.5) -> (249, 4)
  constraints: 16 end point
extrude "Extrusion25" add sketch "Sketch_35" along normal mid plane 85
sketch "Sketch_36" plane through (0, 0, -11.5) normal (0, 0, 1) x (1, 0, 0)
  line L0 (-274, 0) -> (-272.5263, 0)
  line L1 (-272.5263, 0) -> (-265.5981, 4)
  line L2 (-265.5981, 4) -> (-249, 4)
  line L3 (-249, 4) -> (-249, 5.5)
  line L4 (-249, 5.5) -> (-266, 5.5)
  line L5 (-266, 5.5) -> (-272.9282, 1.5)
  line L6 (-272.9282, 1.5) -> (-274, 1.5)
  line L7 (-274, 1.5) -> (-274, 0)
  constraints: 16 end point
extrude "Extrusion26" add sketch "Sketch_36" along normal mid plane 85
sketch "Sketch_37" plane through (0, 5.5, 0) normal (0, 1, 0) x (1, 0, 0)
  arc A0 (-264, -32) -> (-236, -60) centre (-236, -32) ccw
  line L0 (-236, -60) -> (236, -60)
  arc A1 (236, -60) -> (264, -32) centre (236, -32) ccw
  line L1 (264, -32) -> (264, 55)
  arc A2 (264, 55) -> (236, 83) centre (236, 55) ccw
  line L2 (236, 83) -> (-236, 83)
  arc A3 (-236, 83) -> (-264, 55) centre (-236, 55) ccw
  line L3 (-264, 55) -> (-264, -32)
  constraints: 8 end point, 8 point on circle, 4 centre point
extrude "Extrusion27" cut sketch "Sketch_37" against normal blind 1.5
sketch "Sketch_87" plane through (0, 5.5, 0) normal (0, 1, 0) x (1, 0, 0)
  arc A0 (-264, -32) -> (-236, -60) centre (-236, -32) ccw
  line L0 (-236, -60) -> (236, -60)
  arc A1 (236, -60) -> (264, -32) centre (236, -32) ccw
  line L1 (264, -32) -> (264, 55)
  arc A2 (264, 55) -> (236, 83) centre (236, 55) ccw
  line L2 (236, 83) -> (-236, 83)
  arc A3 (-236, 83) -> (-264, 55) centre (-236, 55) ccw
  line L3 (-264, 55) -> (-264, -32)
  circle A4 centre (259, 11.5) radius 2.2
  circle A5 centre (220, -55) radius 2.2
  circle A6 centre (220, 78) radius 2.2
  circle A7 centre (110, -55) radius 2.2
  circle A8 centre (110, 78) radius 2.2
  circle A9 centre (0, -55) radius 2.2
  circle A10 centre (0, 78) radius 2.2
  circle A11 centre (-110, -55) radius 2.2
  circle A12 centre (-110, 78) radius 2.2
  circle A13 centre (-220, -55) radius 2.2
  circle A14 centre (-220, 78) radius 2.2
  arc A15 (-249, -37) -> (-241, -45) centre (-241, -37) ccw
  line L4 (-241, -45) -> (241, -45)
  arc A16 (241, -45) -> (249, -37) centre (241, -37) ccw
  line L5 (249, -37) -> (249, 60)
  arc A17 (249, 60) -> (241, 68) centre (241, 60) ccw
  line L6 (241, 68) -> (-241, 68)
  arc A18 (-241, 68) -> (-249, 60) centre (-241, 60) ccw
  line L7 (-249, 60) -> (-249, -37)
  circle A19 centre (-259, 11.5) radius 2.2
  constraints: 20 centre point, 16 end point, 16 point on circle
extrude "Extrusion28" add sketch "Sketch_87" against normal blind 1.5
sketch "Sketch_106" plane through (0, 0, 12.5) normal (0, 0, 1) x (1, 0, 0)
  line L0 (298.5, 17.5) -> (278.1, 17.5)
  line L1 (278.1, 17.5) -> (278.1, 21.5)
  line L2 (278.1, 21.5) -> (293.1, 21.5)
  line L3 (293.1, 21.5) -> (293.1, 24.5)
  line L4 (293.1, 24.5) -> (298.5, 24.5)
  line L5 (298.5, 24.5) -> (298.5, 17.5)
  line L6 (298.5, 17.5) -> (278.1, 17.5)
  constraints: 14 end point
revolve "Revolution35" add sketch "Sketch_106" angle 360 about axis through (298.5, 17.5, 12.5) along (-1, 0, 0)
ref_plane "FP1_XY" through (0, -0.5, -11.5) normal (0, 1, 0) x (1, 0, 0)
ref_plane "FP1_YZ" through (0, -0.5, -11.5) normal (1, 0, 0) x (0, 0, -1)
ref_plane "FP1_ZX" through (0, -0.5, -11.5) normal (0, 0, -1) x (0, 1, 0)
ref_plane "FP2_XY" through (0, -0.5, -11.5) normal (0, 1, 0) x (1, 0, 0)
ref_plane "FP2_YZ" through (0, -0.5, -11.5) normal (1, 0, 0) x (0, 0, -1)
ref_plane "FP2_ZX" through (0, -0.5, -11.5) normal (0, 0, -1) x (0, 1, 0)
ref_plane "GEHAEUSE_XY" through (0, 300, -105) normal (0, 1, 0) x (1, 0, 0)
ref_plane "GEHAEUSE_YZ" through (0, 300, -105) normal (1, 0, 0) x (0, 0, -1)
ref_plane "GEHAEUSE_ZX" through (0, 300, -105) normal (0, 0, -1) x (0, 1, 0)
ref_plane "MP_XY" through (0, 25, -85) normal (0, 0, -1) x (1, 0, 0)
ref_plane "MP_YZ" through (0, 25, -85) normal (1, 0, 0) x (0, -1, 0)
ref_plane "MP_ZX" through (0, 25, -85) normal (0, -1, 0) x (0, 0, -1)
ref_plane "REVIT_XY" through (0, 0, -105) normal (0, 0, -1) x (-1, 0, 0)
ref_plane "REVIT_YZ" through (0, 0, -105) normal (-1, 0, 0) x (0, 1, 0)
ref_plane "REVIT_ZX" through (0, 0, -105) normal (0, 1, 0) x (0, 0, -1)
ref_plane "SCLM_XY" through (-279.5, 300, 89.75) normal (1, 0, 0) x (0, 0, -1)
ref_plane "SCLM_YZ" through (-279.5, 300, 89.75) normal (0, 0, -1) x (0, 1, 0)
ref_plane "SCLM_ZX" through (-279.5, 300, 89.75) normal (0, 1, 0) x (1, 0, 0)
ref_plane "SCLO_XY" through (-279.5, 537.5, 89.75) normal (1, 0, 0) x (0, 0, -1)
ref_plane "SCLO_YZ" through (-279.5, 537.5, 89.75) normal (0, 0, -1) x (0, 1, 0)
ref_plane "SCLO_ZX" through (-279.5, 537.5, 89.75) normal (0, 1, 0) x (1, 0, 0)
ref_plane "SCLU_XY" through (-279.5, 62.5, 89.75) normal (1, 0, 0) x (0, 0, -1)
ref_plane "SCLU_YZ" through (-279.5, 62.5, 89.75) normal (0, 0, -1) x (0, 1, 0)
ref_plane "SCLU_ZX" through (-279.5, 62.5, 89.75) normal (0, 1, 0) x (1, 0, 0)
ref_plane "SCRM_XY" through (279.5, 300, 89.75) normal (-1, 0, 0) x (0, 0, -1)
ref_plane "SCRM_YZ" through (279.5, 300, 89.75) normal (0, 0, -1) x (0, -1, 0)
ref_plane "SCRM_ZX" through (279.5, 300, 89.75) normal (0, -1, 0) x (-1, 0, 0)
ref_plane "SCRO_XY" through (279.5, 537.5, 89.75) normal (-1, 0, 0) x (0, 0, -1)
ref_plane "SCRO_YZ" through (279.5, 537.5, 89.75) normal (0, 0, -1) x (0, -1, 0)
ref_plane "SCRO_ZX" through (279.5, 537.5, 89.75) normal (0, -1, 0) x (-1, 0, 0)
ref_plane "SCRU_XY" through (279.5, 62.5, 89.75) normal (-1, 0, 0) x (0, 0, -1)
ref_plane "SCRU_YZ" through (279.5, 62.5, 89.75) normal (0, 0, -1) x (0, -1, 0)
ref_plane "SCRU_ZX" through (279.5, 62.5, 89.75) normal (0, -1, 0) x (-1, 0, 0)
ref_plane "to_Abst_tzung_L_XY" through (-250, 25, -76.75) normal (0, 0, 1) x (1, 0, 0)
ref_plane "to_Abst_tzung_L_YZ" through (-250, 25, -76.75) normal (1, 0, 0) x (0, 1, 0)
ref_plane "to_Abst_tzung_L_ZX" through (-250, 25, -76.75) normal (0, 1, 0) x (0, 0, 1)
ref_plane "to_Abst_tzung_R_XY" through (250, 25, -76.75) normal (0, 0, 1) x (1, 0, 0)
ref_plane "to_Abst_tzung_R_YZ" through (250, 25, -76.75) normal (1, 0, 0) x (0, 1, 0)
ref_plane "to_Abst_tzung_R_ZX" through (250, 25, -76.75) normal (0, 1, 0) x (0, 0, 1)
ref_plane "to_Cap_1_XY" through (280, 20, -105) normal (0, 0, 1) x (1, 0, 0)
ref_plane "to_Cap_1_YZ" through (280, 20, -105) normal (1, 0, 0) x (0, 1, 0)
ref_plane "to_Cap_1_ZX" through (280, 20, -105) normal (0, 1, 0) x (0, 0, 1)
ref_plane "to_Cap_2_XY" through (-280, 20, -105) normal (0, 0, 1) x (1, 0, 0)
ref_plane "to_Cap_2_YZ" through (-280, 20, -105) normal (1, 0, 0) x (0, 1, 0)
ref_plane "to_Cap_2_ZX" through (-280, 20, -105) normal (0, 1, 0) x (0, 0, 1)
ref_plane "to_Cap_3_XY" through (280, 580, -105) normal (0, 0, 1) x (1, 0, 0)
ref_plane "to_Cap_3_YZ" through (280, 580, -105) normal (1, 0, 0) x (0, 1, 0)
ref_plane "to_Cap_3_ZX" through (280, 580, -105) normal (0, 1, 0) x (0, 0, 1)
ref_plane "to_Cap_4_XY" through (-280, 580, -105) normal (0, 0, 1) x (1, 0, 0)
ref_plane "to_Cap_4_YZ" through (-280, 580, -105) normal (1, 0, 0) x (0, 1, 0)
ref_plane "to_Cap_4_ZX" through (-280, 580, -105) normal (0, 1, 0) x (0, 0, 1)
ref_plane "to_Plug_XY" through (-283.5, 0, 66) normal (0, 1, 0) x (1, 0, 0)
ref_plane "to_Plug_YZ" through (-283.5, 0, 66) normal (1, 0, 0) x (0, 0, -1)
ref_plane "to_Plug_ZX" through (-283.5, 0, 66) normal (0, 0, -1) x (0, 1, 0)
ref_plane "to_Plug_3_XY" through (250, 600, 16.5) normal (0, 1, 0) x (1, 0, 0)
ref_plane "to_Plug_3_YZ" through (250, 600, 16.5) normal (1, 0, 0) x (0, 0, -1)
ref_plane "to_Plug_3_ZX" through (250, 600, 16.5) normal (0, 0, -1) x (0, 1, 0)
ref_plane "to_Plug_4_XY" through (-250, 600, 16.5) normal (0, 1, 0) x (1, 0, 0)
ref_plane "to_Plug_4_YZ" through (-250, 600, 16.5) normal (1, 0, 0) x (0, 0, -1)
ref_plane "to_Plug_4_ZX" through (-250, 600, 16.5) normal (0, 0, -1) x (0, 1, 0)
ref_plane "to_Plug_1_1_XY" through (255, 0, -60) normal (0, 1, 0) x (1, 0, 0)
ref_plane "to_Plug_1_1_YZ" through (255, 0, -60) normal (1, 0, 0) x (0, 0, -1)
ref_plane "to_Plug_1_1_ZX" through (255, 0, -60) normal (0, 0, -1) x (0, 1, 0)
ref_plane "to_Plug_1_2_XY" through (-255, 0, -60) normal (0, 1, 0) x (1, 0, 0)
ref_plane "to_Plug_1_2_YZ" through (-255, 0, -60) normal (1, 0, 0) x (0, 0, -1)
ref_plane "to_Plug_1_2_ZX" through (-255, 0, -60) normal (0, 0, -1) x (0, 1, 0)